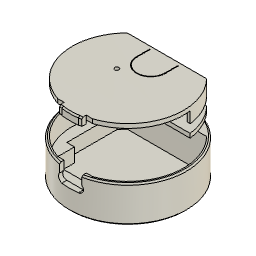
super (Autodesk Fusion 360 design; units mm, degrees)
Autodesk Fusion 360 part; units mm, degrees
sketch "Sketch1" plane through (0, 0, 0) normal (0, 0, 1) x (1, 0, 0)
  circle A0 centre (0, 0) radius 21
  line L0 (-12.5, 15.6125) -> (12.5, 15.6125) construction
  line L1 (12.5, 15.6125) -> (12.5, -4.3875) construction
  line L2 (12.5, -4.3875) -> (-12.5, -4.3875) construction
  line L3 (-12.5, -4.3875) -> (-12.5, 15.6125) construction
  line L4 (-9, 3.1394) -> (9, 3.1394) construction
  line L5 (9, 3.1394) -> (9, -17.8606) construction
  line L6 (9, -17.8606) -> (-9, -17.8606)
  line L7 (-9, -17.8606) -> (-9, 3.1394) construction
  line L8 (9, -4.8606) -> (-9, -4.8606) construction
  circle A1 centre (0, 0) radius 20
  line L9 (0, 1.75) -> (0, 22.5)
  dimension "d1" = 42
  dimension "d5" = 25
  dimension "d6" = 20
  dimension "d7" = 18
  dimension "d8" = 21
  dimension "d12" = 8
  dimension "d13" = -1
  constraint coincident A0.centre A1.centre
  constraint horizontal L0
  constraint vertical L1
  constraint horizontal L2
  constraint vertical L3
  constraint horizontal L4
  constraint vertical L5
  constraint horizontal L6
  constraint vertical L7
  constraint coincident L5 L8.start
  constraint coincident L7 L8.end
  constraint perpendicular L7 L8
  constraint symmetric L5 L7 L9
  constraint coincident L5.end A1
  constraint symmetric L1 L3 L9
  constraint coincident L0.end A1
  measures "d1" diameter of A0
  measures "d5" distance of L0.start L0.end
  measures "d6" distance of L0.start L2.end
  measures "d7" distance of L4.start L4.end
  measures "d8" distance of L4.start L6.end
  measures "d12" distance of L4 L8
extrude "Extrude1" add sketch "Sketch1" along normal blind 13 contours A0 | L6 A1 | L6 A1 makes body 1
chamfer "Chamfer1" distance 0.5 angle 45 1 edges at (-19.5789, -7.5939, 0) on bodies 1
sketch "Sketch2" plane through (0, 0, 13) normal (0, 0, 1) x (-1, 0, 0)
  circle A0 centre (0, 0) radius 21
  circle A1 centre (0, 0) radius 21
  circle A2 centre (0, 0) radius 20
  line L0 (6.245, 19) -> (-6.245, 19)
  line L1 (0, 19) -> (0, 20) construction
  dimension "d9" = -1
  dimension "d63" = 1
  constraint coincident A2 L0.start
  constraint coincident A2 L0.end
  constraint horizontal L0
  constraint midpoint L0 L1.start
  constraint coincident A2 L1.end
  constraint perpendicular L0 L1
  measures "d63" distance of L1.start L1.end
extrude "Extrude2" cut sketch "Sketch2" against normal blind 12 contours A2 L0 picked at (-5.9419, 6.5664) bodies 1
sketch "Sketch3" plane through (0, 0, 1) normal (0, 0, 1) x (-1, 0, 0)
  line L0 (13.2288, 15) -> (-13.2288, 15)
  line L1 (0, 0) -> (0, 19) construction
  line L2 (19.0788, 6) -> (-19.0788, 6)
  line L3 (0, 6) -> (0, -20) construction
  line L4 (14.2829, -14) -> (-14.2829, -14)
  line L5 (13.2288, 15) -> (13.2288, 6)
  line L6 (16, -12) -> (16, 6)
  line L7 (-16, 6) -> (-16, -12)
  line L8 (6.245, 19) -> (-6.245, 19)
  arc A0 (-6.245, 19) -> (6.245, 19) centre (0, 0) ccw
  arc A1 (-6.245, 19) -> (6.245, 19) centre (0, 0) ccw
  line L9 (-6.245, 19) -> (6.245, 19)
  circle A2 centre (0, 0) radius 21
  dimension "d14" = 4
  dimension "d22" = 6
  dimension "d27" = 20
  dimension "d30" = 16
  dimension "d31" = 16
  constraint horizontal L0
  constraint vertical L1
  constraint horizontal L2
  constraint midpoint L2 L3.start
  constraint perpendicular L2 L3
  constraint horizontal L4
  constraint coincident L2 L5.end
  constraint perpendicular L2 L5
  constraint coincident L2 L6.end
  constraint perpendicular L2 L6
  constraint coincident L2 L7.start
  constraint perpendicular L2 L7
  constraint coincident L0.start A0
  constraint coincident L0.end A0
  constraint midpoint L1.end L9
  constraint coincident L2.start A0
  constraint coincident L2.end A0
  constraint coincident L4.end A0
  constraint coincident L4.start A1
  constraint coincident L3.end A0
  constraint coincident L6.start A1
  constraint coincident L7.end A1
  measures "d14" distance of L0 L1.end
  measures "d22" distance of L3.end L4
  measures "d27" distance of L2 L4
  measures "d30" distance of L1.start L6
  measures "d31" distance of L1.start L7
extrude "Extrude3" add sketch "Sketch3" along normal blind 5 contours L0 L8 A0 A1 L9 bodies 1
sketch "Sketch4" plane through (0, 0, 13) normal (0, 0, 1) x (-1, 0, 0)
  circle A0 centre (0, 0) radius 21
  line L0 (0, 0) -> (0, 21) construction
  line L1 (0, 21) -> (-4.5, 21)
  line L2 (0, 21) -> (4.5, 21)
  arc A1 (-6.245, 19) -> (6.245, 19) centre (0, 0) ccw
  line L3 (-6.245, 19) -> (6.245, 19)
  line L4 (4.5, 21) -> (4.5, 19)
  line L5 (-4.5, 21) -> (-4.5, 19)
  dimension "d17" = 4.5
  dimension "d18" = 4.5
  constraint coincident A0.centre L0.start
  constraint coincident A0 L0.end
  constraint vertical L0
  constraint perpendicular L0 L1
  constraint perpendicular L0 L2
  constraint coincident L3 L4.end
  constraint perpendicular L3 L4
  constraint coincident L3 L5.end
  constraint perpendicular L3 L5
  measures "d17" distance of L0.end L1.end
  measures "d18" distance of L0.end L2.end
extrude "Extrude4" cut sketch "Sketch4" against normal blind 5.8 contours A0 L3 L4 L5 | A0 L2 L4 | A0 L1 L5 bodies 1
extrude "Extrude16" add sketch "Sketch4" against normal blind 2.8 contours A0 L3 L4 L5 bodies 1
extrude "Extrude5" add sketch "Sketch3" along normal blind 12 contours L4 A0 A1 bodies 1
extrude "Extrude6" add sketch "Sketch3" along normal blind 5 contours L2 L5 A0 A1 | L2 L6 A0 A1 | L2 L7 A0 A1 bodies 1
fillet "Fillet1" radius 1.5 4 edges at (-4.5, -19.7561, 7.2) (-4.5, -19.7561, 10.2) (4.5, -19.7561, 7.2) (4.5, -19.7561, 10.2) on bodies 1
ref_plane "WorkPlane1" through (0, 0, 21) normal (0, 0, 1) x (1, 0, 0)
sketch "Sketch5" plane through (0, 0, 21) normal (0, 0, 1) x (1, 0, 0)
  line L0 (16, -6) -> (16, 12)
  arc A0 (16, 12) -> (14.2829, 14) centre (0, 0) ccw
  line L1 (19.0788, -6) -> (16, -6)
  arc A1 (-16, 12) -> (-13.2288, -15) centre (0, 0) ccw
  line L2 (-13.2288, -6) -> (-16, -6)
  arc A2 (19.0788, -6) -> (16, 12) centre (0, 0) ccw
  line L3 (16, 12) -> (16, -6)
  line L4 (16, -6) -> (19.0788, -6)
  line L5 (-19.8431, 2.5) -> (19.8431, 2.5)
  line L6 (14.2829, 14) -> (-14.2829, 14)
  arc A3 (13.2288, -15) -> (19.0788, -6) centre (0, 0) ccw
  circle A4 centre (0, 0) radius 21
  line L7 (6.245, -19) -> (-6.245, -19)
  arc A5 (-14.2829, 14) -> (-6.245, -19) centre (0, 0) ccw
  line L8 (-14.2829, 14) -> (14.2829, 14)
  arc A6 (6.245, -19) -> (14.2829, 14) centre (0, 0) ccw
  arc A7 (-14.2829, 14) -> (-16, 12) centre (0, 0) ccw
  line L9 (-16, 12) -> (-16, -6)
  line L10 (-16, -6) -> (-13.2288, -6)
  line L11 (-13.2288, -6) -> (-13.2288, -15)
  line L12 (-13.2288, -15) -> (13.2288, -15)
  line L13 (-13.2288, -15) -> (-13.2288, -6)
  line L14 (-16, -6) -> (-16, 12)
  constraint coincident A1 L5.start
  constraint horizontal L5
extrude "Extrude7" add sketch "Sketch5" along normal blind 1.5 separate body contours L0 A0 L3 L5 L6 A5 L8 A6 A7 L9 L14 | L0 A2 L3 L5 A6 | A1 L5 A5 L9 L14 makes body 2
sketch "Sketch6" plane through (0, 0, 22.5) normal (0, 0, 1) x (-1, 0, 0)
  line L0 (0, -2.5) -> (0, -14) construction
  line L1 (-3, -5.25) -> (3, -5.25)
  line L2 (3, -5.25) -> (3, -11.25)
  line L3 (3, -11.25) -> (-3, -11.25)
  line L4 (-3, -11.25) -> (-3, -5.25)
  line L5 (-3, -5.25) -> (3, -11.25) construction
  line L6 (3, -5.25) -> (-3, -11.25) construction
  arc A0 (-19.8431, -2.5) -> (-14.2829, -14) centre (0, 0) ccw
  line L7 (19.8431, -2.5) -> (-19.8431, -2.5)
  arc A1 (14.2829, -14) -> (19.8431, -2.5) centre (0, 0) ccw
  line L8 (-14.2829, -14) -> (14.2829, -14)
  point P0 (0, -8.25)
  dimension "d36" = 6
  dimension "d37" = 6
  constraint horizontal L1
  constraint perpendicular L1 L2
  constraint parallel L1 L3
  constraint parallel L2 L4
  constraint coincident L5 P0
  constraint coincident L6 P0
  constraint coincident L0 P0
  constraint midpoint L0 P0
  measures "d36" distance of L2.end L3.end
  measures "d37" distance of L1.end L2.end
extrude "Extrude8" cut sketch "Sketch6" against normal blind 1 contours L1 L2 L3 L4 bodies 2
ref_plane "WorkPlane2" through (0, 8.25, 29.5) normal (0, 0, 1) x (1, 0, 0)
sketch "Sketch7" plane through (0, 0, 29.5) normal (0, 0, 1) x (1, 0, 0)
  line L0 (-14.2829, 14) -> (14.2829, 14)
  arc A0 (-14.2829, 14) -> (-6.245, -19) centre (0, 0) ccw
  line L1 (6.245, -19) -> (-6.245, -19)
  arc A1 (6.245, -19) -> (14.2829, 14) centre (0, 0) ccw
extrude "Extrude9" add sketch "Sketch7" along normal blind 1.5 separate body makes body 3
sketch "Sketch10" plane through (0, 0, 13) normal (0, 0, 1) x (-1, 0, 0)
  line L0 (0, -14) -> (0, -21) construction
  circle A0 centre (0, -17.5) radius 1
  circle A1 centre (0, 0) radius 21
  line L1 (-6.245, 19) -> (6.245, 19)
  arc A2 (14.2829, -14) -> (6.245, 19) centre (0, 0) ccw
  line L2 (14.2829, -14) -> (-14.2829, -14)
  arc A3 (-6.245, 19) -> (-14.2829, -14) centre (0, 0) ccw
  dimension "d53" = 2
  constraint midpoint L0 A0.centre
  constraint vertical L0
  measures "d53" diameter of A0
extrude "Extrude13" cut sketch "Sketch10" against normal blind 23 contours A0 bodies 1
sketch "Sketch11" plane through (0, 0, 29.5) normal (0, 0, -1) x (1, 0, 0)
  line L0 (3.5, 18.6748) -> (3.5, 19.6914)
  spline S0 degree 3 poles (2.8571, 19.7949) (3.0365, 19.769) (3.2303, 19.7382) (3.4058, 19.7079) (3.4377, 19.7024) (3.4691, 19.6968) (3.5, 19.6914) knots -0.227788 -0.227788 -0.227788 -0.227788 -0.170413 -0.170413 -0.170413 -0.160012 -0.160012 -0.160012 -0.160012
  arc A0 (2.8571, 19.7949) -> (-2.8571, 19.7949) centre (0, 0) ccw
  spline S1 degree 3 poles (-3.5, 19.6914) (-3.4691, 19.6968) (-3.4377, 19.7024) (-3.4058, 19.7079) (-3.2303, 19.7382) (-3.0365, 19.769) (-2.8571, 19.7949) knots 0.160012 0.160012 0.160012 0.160012 0.170413 0.170413 0.170413 0.227788 0.227788 0.227788 0.227788
  line L1 (-3.5, 19.6914) -> (-3.5, 18.6748)
  arc A1 (-3.5, 18.6748) -> (-13.8564, -13) centre (0, 0) ccw
  line L2 (-13.8564, -13) -> (13.8564, -13)
  arc A2 (13.8564, -13) -> (3.5, 18.6748) centre (0, 0) ccw
  line L3 (-14.2829, -14) -> (14.2829, -14)
  line L4 (19.8431, -2.5) -> (-19.8431, -2.5)
  arc A3 (14.2829, -14) -> (19.8431, -2.5) centre (0, 0) ccw
  arc A4 (-19.8431, -2.5) -> (-14.2829, -14) centre (0, 0) ccw
  line L5 (-14.2829, -14) -> (14.2829, -14)
  arc A5 (-6.245, 19) -> (-14.2829, -14) centre (0, 0) ccw
  arc A6 (14.2829, -14) -> (6.245, 19) centre (0, 0) ccw
  line L6 (6.245, 19) -> (-6.245, 19)
  constraint tangent A0 S1
  constraint tangent S0 A0
extrude "Extrude14" add sketch "Sketch11" along normal blind 4 contours A1 L2 A2 L3 L4 A3 A4 L5 A5 A6 bodies 3
sketch "Sketch9" plane through (0, 0, 29.5) normal (0, 0, -1) x (1, 0, 0)
  arc A0 (-6.245, 19) -> (-19.8431, -2.5) centre (0, 0) ccw
  arc A1 (19.8431, -2.5) -> (6.245, 19) centre (0, 0) ccw
  line L0 (6.245, 19) -> (-6.245, 19)
  line L1 (3, -11.25) -> (-3, -11.25)
  line L2 (-3, -11.25) -> (-3, -5.25)
  line L3 (-3, -5.25) -> (3, -5.25)
  line L4 (3, -5.25) -> (3, -11.25)
  line L5 (3, -11.25) -> (-3, -5.25) construction
  arc A2 (5, -8.25) -> (-5, -8.25) centre (0, -8.25) ccw
  line L6 (5, -8.25) -> (-5, -8.25)
  line L7 (5, -8.25) -> (5, -13)
  line L8 (-5, -8.25) -> (-5, -13)
  line L9 (-5.2, -8.25) -> (-5.2, -13)
  arc A3 (5.2, -8.25) -> (-5.2, -8.25) centre (0, -8.25) ccw
  line L10 (5.2, -8.25) -> (5.2, -13)
  line L11 (5, -13) -> (-5, -13)
  line L12 (18.8348, -2.5) -> (19.8431, -2.5)
  line L13 (-19.8431, -2.5) -> (-18.8348, -2.5)
  arc A4 (-18.8348, -2.5) -> (-13.8564, -13) centre (0, 0) ccw
  line L14 (-13.8564, -13) -> (13.8564, -13)
  arc A5 (13.8564, -13) -> (18.8348, -2.5) centre (0, 0) ccw
  point P0 (0, -8.25)
  dimension "d84" = 5
  dimension "d85" = 0.2
  constraint coincident L1.start L4.end
  constraint coincident L2.end L3.start
  constraint midpoint L5 P0
  constraint coincident P0 A2.centre
  constraint midpoint P0 L6
  constraint horizontal L6
  constraint tangent A2 L7
  constraint tangent A2 L8
  constraint perpendicular L8 L11
  constraint coincident L8.end L14
  constraint coincident L10.end L11
  measures "d84" radius of A2
extrude "Extrude15" cut sketch "Sketch9" against normal blind 0.6 contours L1 L2 L4 L6 L7 L8 L11 L14 | L2 L3 L4 A2 L6 | L1 L2 L4 L6 | L2 L3 L4 L6 bodies 3
extrude "Extrude21" cut sketch "Sketch9" against normal blind 1.5 contours A2 L7 L8 L9 A3 L10 L14 bodies 3
chamfer "Chamfer3" distance 0.5 angle 45 1 edges at (19.5789, 7.5939, 13) on bodies 1
sketch "Sketch12" plane through (0, 0, 13) normal (0, 0, 1) x (-1, 0, 0)
  line L0 (-6.245, 19) -> (6.245, 19)
  arc A0 (14.2829, -14) -> (6.245, 19) centre (0, 0) ccw
  line L1 (14.2829, -14) -> (-14.2829, -14)
  arc A1 (-6.245, 19) -> (-14.2829, -14) centre (0, 0) ccw
  circle A2 centre (0, -17.5) radius 1
  circle A3 centre (0, 0) radius 20.5
  line L2 (-3, 20.7846) -> (-3, 19)
  line L3 (-3, 19) -> (3, 19)
  line L4 (3, 19) -> (3, 20.7846)
  arc A4 (3, 20.7846) -> (-3, 20.7846) centre (0, 0) ccw
  line L5 (3, 19) -> (4, 19)
  line L6 (4, 19) -> (4, 20.7846)
  line L7 (4, 20.7846) -> (3, 20.7846)
  line L8 (3, 20.7846) -> (3, 19)
  line L9 (-3, 19) -> (-4, 19)
  line L10 (-4, 19) -> (-4, 20.7846)
  line L11 (-4, 20.7846) -> (-3, 20.7846)
  line L12 (-3, 20.7846) -> (-3, 19)
  dimension "d67" = 1
  dimension "d68" = 1
  constraint horizontal L5
  constraint vertical L6
  constraint horizontal L7
  constraint vertical L8
  constraint coincident L3.end L4.start
  constraint coincident L4.end A4.start
  constraint horizontal L9
  constraint vertical L10
  constraint horizontal L11
  constraint vertical L12
  constraint coincident L2.end L3.start
  constraint coincident L2.start A4.end
  measures "d67" distance of L6.end L4.end
  measures "d68" distance of L2.end L9.end
extrude "Extrude17" cut sketch "Sketch12" against normal blind 4 contours L0 A3 L2 L9 L10 L12 | L0 A3 L2 L3 L4 L8 L12 | A3 L2 L10 L11 L12 | L0 A3 L4 L5 L6 L8 | A3 L2 L4 A4 L8 L12 | A3 L4 L6 L7 L8 bodies 1
sketch "Sketch13" plane through (0, 0, 31) normal (0, 0, 1) x (-1, 0, 0)
  arc A0 (14.2829, -14) -> (6.245, 19) centre (0, 0) ccw
  line L0 (6.245, 19) -> (-6.245, 19)
  arc A1 (-6.245, 19) -> (-14.2829, -14) centre (0, 0) ccw
  line L1 (-14.2829, -14) -> (14.2829, -14)
  line L2 (4, 20.106) -> (4, 19)
  line L3 (4, 20.6155) -> (4, 20.106)
  line L4 (-4, 19) -> (-4, 20.106)
  line L5 (-4, 20.106) -> (-4, 20.6155)
  arc A2 (3, 20.7846) -> (-3, 20.7846) centre (0, 0) ccw
  spline S0 degree 3 poles (4.5, 20.5122) (4.5, 20.5122) (4.4623, 20.5206) (4.31, 20.5531) (4.1954, 20.5771) (3.9304, 20.6294) (3.7613, 20.6613) (3.3908, 20.7253) (3.1893, 20.7573) (3, 20.7846) knots 0 0 0 0 0.056519 0.056519 0.113038 0.113038 0.170413 0.170413 0.227788 0.227788 0.227788 0.227788
  spline S1 degree 3 poles (-3, 20.7846) (-3.1893, 20.7573) (-3.3908, 20.7253) (-3.7613, 20.6613) (-3.9304, 20.6294) (-4.1954, 20.5771) (-4.31, 20.5531) (-4.4623, 20.5206) (-4.5, 20.5122) (-4.5, 20.5122) knots -0.227788 -0.227788 -0.227788 -0.227788 -0.170413 -0.170413 -0.113038 -0.113038 -0.056519 -0.056519 0 0 0 0
  line L6 (5.2, -8.25) -> (5.2, -13)
  line L7 (5.2, -13) -> (5, -13)
  line L8 (5, -13) -> (5, -8.25)
  arc A3 (5, -8.25) -> (-5, -8.25) centre (0, -8.25) ccw
  line L9 (-5, -8.25) -> (-5, -13)
  line L10 (-5, -13) -> (-5.2, -13)
  line L11 (-5.2, -13) -> (-5.2, -8.25)
  arc A4 (5.2, -8.25) -> (-5.2, -8.25) centre (0, -8.25) ccw
extrude "Extrude18" add sketch "Sketch13" against normal blind 2.7 contours L0 L2 L3 L4 L5 A2 S0 S1 bodies 3
chamfer "Chamfer4" distance 0.5 angle 45 3 edges at (0, -21, 31) (3.5332, -20.7006, 31) (-3.5332, -20.7006, 31) on bodies 3
sketch "Sketch14" plane through (0, 0, 31) normal (0, 0, 1) x (-1, 0, 0)
  spline S0 degree 3 poles (-4, 20.106) (-3.9261, 20.1207) (-3.8431, 20.1368) (-3.6569, 20.1714) (-3.5554, 20.1896) (-3.4491, 20.2078) (-3.3647, 20.2221) (-3.2771, 20.2365) (-3.1016, 20.2642) (-3.0137, 20.2775) (-2.9286, 20.2897) knots 0.108155 0.108155 0.108155 0.108155 0.141485 0.141485 0.174814 0.174814 0.174814 0.201301 0.201301 0.227788 0.227788 0.227788 0.227788
  line L0 (-4, 20.106) -> (-4, 19)
  line L1 (-4, 19) -> (-6.245, 19)
  arc A0 (-6.245, 19) -> (-14.2829, -14) centre (0, 0) ccw
  line L2 (-14.2829, -14) -> (14.2829, -14)
  arc A1 (14.2829, -14) -> (6.245, 19) centre (0, 0) ccw
  line L3 (6.245, 19) -> (4, 19)
  line L4 (4, 19) -> (4, 20.106)
  spline S1 degree 3 poles (2.9286, 20.2897) (3.0137, 20.2775) (3.1016, 20.2642) (3.2771, 20.2365) (3.3647, 20.2221) (3.4491, 20.2078) (3.5554, 20.1896) (3.6569, 20.1714) (3.8431, 20.1368) (3.9261, 20.1207) (4, 20.106) knots -0.227788 -0.227788 -0.227788 -0.227788 -0.201301 -0.201301 -0.174814 -0.174814 -0.174814 -0.141485 -0.141485 -0.108155 -0.108155 -0.108155 -0.108155
  arc A2 (2.9286, 20.2897) -> (-2.9286, 20.2897) centre (0, 0) ccw
  line L5 (4, 19) -> (-4, 19) construction
  line L6 (0, 19) -> (0, -1) construction
  line L7 (0, -1) -> (5, -1) construction
  circle A3 centre (5, -1) radius 0.75
  line L8 (5.2, -8.25) -> (5.2, -13)
  line L9 (5.2, -13) -> (5, -13)
  line L10 (5, -13) -> (5, -8.25)
  arc A4 (5, -8.25) -> (-5, -8.25) centre (0, -8.25) ccw
  line L11 (-5, -8.25) -> (-5, -13)
  line L12 (-5, -13) -> (-5.2, -13)
  line L13 (-5.2, -13) -> (-5.2, -8.25)
  arc A5 (5.2, -8.25) -> (-5.2, -8.25) centre (0, -8.25) ccw
  dimension "d76" = 20
  dimension "d77" = 5
  dimension "d78" = 1.5
  constraint coincident L3.end L4.start
  constraint coincident L0.end L1.start
  constraint midpoint L5 L6.start
  constraint perpendicular L5 L6
  constraint perpendicular L6 L7
  constraint coincident L7.end A3.centre
  measures "d76" distance of L6.start L6.end
  measures "d77" distance of L6.end L7.end
  measures "d78" diameter of A3
extrude "Extrude19" cut sketch "Sketch14" against normal blind 1.5 contours A3 bodies 3
sketch "Sketch15" plane through (0, 0, 29.5) normal (0, 0, -1) x (1, 0, 0)
  circle A0 centre (-5, -1) radius 0.75
  line L0 (18.8348, -2.5) -> (19.8431, -2.5)
  arc A1 (19.8431, -2.5) -> (6.245, 19) centre (0, 0) ccw
  line L1 (6.245, 19) -> (4, 19)
  line L2 (4, 19) -> (-4, 19)
  line L3 (-4, 19) -> (-6.245, 19)
  arc A2 (-6.245, 19) -> (-19.8431, -2.5) centre (0, 0) ccw
  line L4 (-19.8431, -2.5) -> (-18.8348, -2.5)
  arc A3 (-18.8348, -2.5) -> (-13.8564, -13) centre (0, 0) ccw
  line L5 (5.2, -13) -> (13.8564, -13)
  arc A4 (13.8564, -13) -> (18.8348, -2.5) centre (0, 0) ccw
  circle A5 centre (-5, -1) radius 0.75
  circle A6 centre (-5, -1) radius 1.3
  line L6 (-13.8564, -13) -> (-5.2, -13)
  line L7 (-5.2, -13) -> (-5.2, -8.25)
  arc A7 (5.2, -8.25) -> (-5.2, -8.25) centre (0, -8.25) ccw
  line L8 (5.2, -8.25) -> (5.2, -13)
  dimension "d81" = 2.6
  constraint concentric A5 A6
  measures "d81" diameter of A6
extrude "Extrude20" add sketch "Sketch15" along normal blind 2 contours A6 bodies 3
equation "d61 = -5.8 mm + 3 mm"
